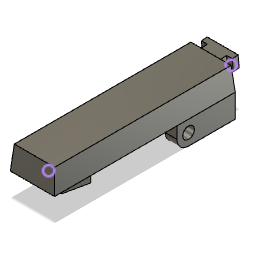
BlackKey (Autodesk Fusion 360 design; units mm, degrees)
Autodesk Fusion 360 part; units mm, degrees
note: some values were not read from the file. Set by a fixed rule: which sketch regions a step uses.
sketch "Sketch1" plane through (0, 0, 0) normal (0, 1, 0) x (1, 0, 0)
  line L0 (-2.54, 0) -> (7.112, 0)
  line L1 (7.112, 0) -> (7.112, -40.64)
  line L2 (7.112, -40.64) -> (-2.54, -40.64)
  line L3 (-2.54, -40.64) -> (-2.54, 0)
  dimension "d1" = 9.652
  dimension "d2" = 40.64
  constraint horizontal L0
  constraint vertical L1
  constraint horizontal L2
  constraint vertical L3
  measures "d1" distance of L0.start L0.end
  measures "d2" distance of L0.end L1.end
extrude "Extrude1" add sketch "Sketch1" along normal blind 5.08 draft -5
sketch "Sketch8" plane through (0, 0, 0) normal (0, -1, 0) x (1, 0, 0)
  line L0 (7.112, 40.64) -> (-2.54, 40.64)
  line L1 (-2.54, 40.64) -> (-2.54, 0)
  line L2 (-2.54, 0) -> (7.112, 0)
  line L3 (7.112, 0) -> (7.112, 40.64)
  line L4 (4.572, 2.54) -> (0, 2.54)
  line L5 (0, 2.54) -> (0, 38.1)
  line L6 (0, 38.1) -> (4.572, 38.1)
  line L7 (4.572, 38.1) -> (4.572, 2.54)
  line L8 (7.112, 0) -> (4.572, 0)
  line L9 (4.572, 0) -> (4.572, 12.7)
  line L10 (4.572, 12.7) -> (7.112, 12.7)
  line L11 (7.112, 12.7) -> (7.112, 0)
  line L12 (0, 0) -> (-2.54, 0)
  line L13 (-2.54, 0) -> (-2.54, 12.7)
  line L14 (-2.54, 12.7) -> (0, 12.7)
  line L15 (0, 12.7) -> (0, 0)
  line L16 (4.572, 0) -> (0, 0)
  line L17 (0, 0) -> (0, 2.54)
  line L18 (0, 2.54) -> (4.572, 2.54)
  line L19 (4.572, 2.54) -> (4.572, 0)
  dimension "d48" = 2.54
  dimension "d49" = 2.54
  dimension "d50" = 2.54
  dimension "d51" = 2.54
  dimension "d52" = 12.7
  dimension "d53" = 12.7
  constraint horizontal L4
  constraint vertical L5
  constraint horizontal L6
  constraint vertical L7
  constraint horizontal L8
  constraint vertical L9
  constraint horizontal L10
  constraint vertical L11
  constraint coincident L7 L9.end
  constraint coincident L2.end L3.start
  constraint horizontal L12
  constraint vertical L13
  constraint horizontal L14
  constraint vertical L15
  constraint coincident L1 L13.end
  constraint coincident L12.start L15.end
  constraint horizontal L16
  constraint vertical L17
  constraint horizontal L18
  constraint vertical L19
  measures "d48" distance of L0 L6
  measures "d49" distance of L2 L4
  measures "d50" distance of L1 L5
  measures "d51" distance of L3 L7
  measures "d52" distance of L2.end L10.end
  measures "d53" distance of L1.end L13.end
extrude "Extrude8" add sketch "Sketch8" along normal blind 5.08 contours L2 L3 L7 L8 L9 L10 L11 L19 | L1 L2 L5 L12 L13 L14 L15 L17
sketch "Sketch9" plane through (0, 0, 0) normal (0, 0.087156, -0.996195) x (-1, 0, 0)
  line L0 (2.0956, 5.0994) -> (-6.6676, 5.0994)
  line L1 (-6.6676, 5.0994) -> (-7.112, 0)
  line L2 (-7.112, 0) -> (-4.572, 0)
  line L3 (2.54, 0) -> (2.0956, 5.0994)
  line L4 (-6.8898, 2.5497) -> (-6.6676, 5.0994)
  line L5 (-6.6676, 5.0994) -> (2.0956, 5.0994)
  line L6 (2.0956, 5.0994) -> (2.3178, 2.5497)
  line L7 (-6.8898, 2.5497) -> (2.3178, 2.5497)
  line L8 (-4.572, 0) -> (0, 0)
  line L9 (0, 0) -> (2.54, 0)
  constraint midpoint L1 L4.start
  constraint coincident L0.end L1.start
  constraint coincident L0.start L3.end
  constraint midpoint L3 L6.end
extrude "Extrude9" add sketch "Sketch9" along normal blind 2.54 contours L0 L1 L3 L4 L5 L6 L7
sketch "Sketch13" plane through (7.112, 0, 0) normal (1, 0, 0) x (0, 0, -1)
  line L0 (-12.7, -5.08) -> (0, -5.08)
  line L1 (0, -5.08) -> (0, 0)
  line L2 (0, 0) -> (-12.7, 0)
  line L3 (-12.7, 0) -> (-12.7, -5.08)
  circle A0 centre (-10.16, -2.54) radius 1.27
  line L4 (0, -2.54) -> (-8.89, -2.54)
  line L5 (-11.43, -2.54) -> (-12.7, -2.54)
  line L6 (-10.16, -3.81) -> (-10.16, -5.08)
  constraint coincident L0 L6.end
  constraint midpoint L1 L4.start
  constraint coincident L3 L5.end
  constraint perpendicular L3 L4
  constraint coincident A0 L5.start
  constraint collinear L4 L5
  constraint coincident A0 L6.start
  constraint coincident A0 L4.end
extrude "Extrude12" cut sketch "Sketch13" against normal blind 20.32 contours A0
sketch "Sketch14" plane through (0, 0, 0) normal (0, -1, 0) x (1, 0, 0)
  line L0 (0, 12.7) -> (0, 0)
  line L1 (0, 0) -> (4.572, 0)
  line L2 (4.572, 0) -> (4.572, 12.7)
  line L3 (4.572, 12.7) -> (7.112, 12.7)
  line L4 (7.112, 12.7) -> (7.112, 40.64)
  line L5 (7.112, 40.64) -> (-2.54, 40.64)
  line L6 (-2.54, 40.64) -> (-2.54, 12.7)
  line L7 (-2.54, 12.7) -> (0, 12.7)
  line L8 (-2.54, 12.7) -> (0, 12.7)
  line L9 (-2.54, 40.64) -> (-2.54, 38.1)
  line L10 (0, 12.7) -> (0, 39.37)
  line L11 (0, 39.37) -> (4.9434, 39.37)
  line L12 (4.9434, 39.37) -> (4.572, 12.7)
  line L13 (0, 12.7) -> (4.572, 12.7)
  dimension "d72" = 2.54
  dimension "d73" = 2.54
  dimension "d74" = 26.67
  constraint coincident L6.end L7.start
  constraint perpendicular L6 L8
  constraint coincident L5.end L6.start
  constraint perpendicular L5 L9
  constraint coincident L0.start L7.end
  constraint perpendicular L8 L10
  constraint perpendicular L10 L11
  constraint coincident L2.end L3.start
  measures "d72" distance of L6.end L0.start
  measures "d73" distance of L5.end L9.end
  measures "d74" distance of L0.start L10.end
extrude "Extrude13" cut sketch "Sketch14" against normal blind 3.81 contours L10 L11 L12 L13
sketch "Sketch15" plane through (0, 0, 0) normal (0, -1, 0) x (1, 0, 0)
  line L0 (4.572, 12.7) -> (0, 12.7)
  line L1 (0, 12.7) -> (0, 0)
  line L2 (0, 0) -> (4.572, 0)
  line L3 (4.572, 0) -> (4.572, 12.7)
  line L4 (0, 0) -> (0, 2.54)
  line L5 (0, 2.54) -> (4.572, 2.54)
  line L6 (4.572, 2.54) -> (4.572, 12.7)
  line L7 (4.572, 12.7) -> (0, 12.7)
  line L8 (0, 12.7) -> (0, 2.54)
  dimension "d77" = 2.54
  constraint coincident L1.end L2.start
  constraint perpendicular L2 L4
  constraint horizontal L5
  constraint vertical L6
  constraint horizontal L7
  constraint vertical L8
  constraint coincident L0.start L3.end
  measures "d77" distance of L1.end L4.end
extrude "Extrude14" cut sketch "Sketch15" against normal blind 2.54 contours L0 L1 L3 L5 L6 L7 L8
extrude "Extrude15" cut 1 faces at (1.524, 2.54, 5.9267) along direction (0, 1, 0) blind 1.27
sketch "Sketch16" plane through (7.112, 0, 0) normal (1, 0, 0) x (0, 0, -1)
  circle A0 centre (-10.16, -2.54) radius 1.27
  line L0 (0, 0) -> (-12.7, 0)
  line L1 (-12.7, 0) -> (-12.7, -5.08)
  line L2 (-12.7, -5.08) -> (0, -5.08)
  line L3 (0, -5.08) -> (0, 0)
  line L4 (-12.7, -2.54) -> (-12.7, -5.08)
  line L5 (-10.16, -5.08) -> (-12.7, -5.08)
  arc A1 (-12.7, -2.54) -> (-10.16, -5.08) centre (-10.16, -2.54) ccw
  constraint concentric A0 A1
  constraint tangent L2 A1
  constraint midpoint L1 L4.start
  constraint coincident L1.end L2.start
  constraint tangent L5 A1
extrude "Extrude16" cut sketch "Sketch16" against normal blind 10.414 contours L1 L2 L4 L5 A1
sketch "Sketch17" plane through (0, 0, 0) normal (0, -1, 0) x (1, 0, 0)
  line L0 (0, 12.7) -> (0, 39.37)
  line L1 (0, 39.37) -> (4.9434, 39.37)
  line L2 (4.9434, 39.37) -> (4.572, 12.7)
  line L3 (4.572, 12.7) -> (7.112, 12.7)
  line L4 (7.112, 12.7) -> (7.112, 40.64)
  line L5 (7.112, 40.64) -> (-2.54, 40.64)
  line L6 (-2.54, 40.64) -> (-2.54, 12.7)
  line L7 (-2.54, 12.7) -> (0, 12.7)
  line L8 (0, 39.37) -> (-1.27, 39.37)
  line L9 (-1.27, 39.37) -> (-1.27, 12.7)
  line L10 (-1.27, 12.7) -> (0, 12.7)
  line L11 (0, 12.7) -> (0, 39.37)
  constraint horizontal L8
  constraint vertical L9
  constraint horizontal L10
  constraint vertical L11
  constraint midpoint L7 L9.end
  constraint coincident L0.end L1.start
extrude "Extrude17" cut sketch "Sketch17" against normal blind 3.81 contours L0 L7 L8 L9 L10 L11
extrude "Extrude18" cut 1 faces at (4.8196, 1.27, 30.48) along direction (0.999903, 0, -0.013923) blind 1.27
sketch "Sketch18" plane through (0, 0, 0) normal (0, 1, 0) x (1, 0, 0)
extrude "Extrude19" add 1 faces at (1.2245, 3.81, 30.48) along direction (0, -1, 0) blind 3.81
sketch "Sketch19" plane through (0, 5.08, 0.4444) normal (0, 0.996195, 0.087156) x (1, 0, 0)
  line L0 (-2.0956, 0) -> (6.6676, 0)
  line L1 (6.6676, 0) -> (6.6676, 2.54)
  line L2 (6.6676, 2.54) -> (-2.0956, 2.54)
  line L3 (-2.0956, 2.54) -> (-2.0956, 0)
  line L4 (2.286, 2.54) -> (-1.0795, 2.54)
  line L5 (2.286, 2.54) -> (5.6642, 2.54)
  line L6 (-1.0795, 2.54) -> (-1.0795, 1.27)
  line L7 (-1.0795, 1.27) -> (0.1905, 1.27)
  line L8 (0.1905, 1.27) -> (0.1905, 0)
  line L9 (5.6642, 2.54) -> (5.6642, 1.27)
  line L10 (5.6642, 1.27) -> (4.3942, 1.27)
  line L11 (4.3942, 1.27) -> (4.3942, 0)
  line L12 (0.1905, 0) -> (4.3942, 0)
  line L13 (4.3942, 0) -> (7.366, 0)
  line L14 (7.366, 0) -> (7.366, 2.54)
  line L15 (7.366, 2.54) -> (5.6642, 2.54)
  line L16 (-1.0795, 2.54) -> (-2.794, 2.54)
  line L17 (-2.794, 2.54) -> (-2.794, 0)
  line L18 (-2.794, 0) -> (0.1905, 0)
  dimension "d91" = 3.3655
  dimension "d92" = 3.3782
  dimension "d93" = 1.27
  dimension "d94" = 1.27
  dimension "d95" = 1.27
  dimension "d96" = 1.27
  constraint midpoint L2 L4.start
  constraint parallel L2 L4
  constraint parallel L2 L5
  constraint perpendicular L2 L6
  constraint perpendicular L6 L7
  constraint coincident L0 L8.end
  constraint perpendicular L0 L8
  constraint perpendicular L5 L9
  constraint perpendicular L9 L10
  constraint coincident L0 L11.end
  constraint perpendicular L0 L11
  constraint perpendicular L1 L13
  constraint perpendicular L0 L14
  constraint perpendicular L6 L16
  constraint perpendicular L16 L17
  constraint perpendicular L8 L18
  measures "d91" distance of L4.start L4.end
  measures "d92" distance of L4.start L5.end
  measures "d93" distance of L4.end L6.end
  measures "d94" distance of L6.end L7.end
  measures "d95" distance of L5.end L9.end
  measures "d96" distance of L9.end L10.end
extrude "Extrude20" cut sketch "Sketch19" against normal blind 5.08 contours L0 L2 L3 L6 L7 L8 L16 L18 | L3 L16 L17 L18 | L0 L1 L2 L9 L10 L11 L13 L15 | L1 L13 L14 L15
sketch "Sketch21" plane through (7.058, 0.6175, 0) normal (0.996195, 0.087156, 0) x (0, 0, -1)
  line L0 (-40.1956, 4.4796) -> (-40.64, -0.6199)
  line L1 (-40.64, -0.6199) -> (-12.7, -0.6199)
  line L2 (-12.7, -0.6199) -> (0, -0.6199)
  line L3 (0, -0.6199) -> (-0.4444, 4.4796)
sketch "Sketch22" plane through (0, 0, 0) normal (0, -1, 0) x (1, 0, 0)
  line L0 (4.572, 12.7) -> (7.112, 12.7)
  line L1 (7.112, 12.7) -> (7.112, 40.64)
  line L2 (7.112, 40.64) -> (-2.54, 40.64)
  line L3 (-2.54, 40.64) -> (-2.54, 12.7)
  line L4 (-2.54, 12.7) -> (0, 12.7)
  line L5 (0, 12.7) -> (0, 0)
  line L6 (0, 0) -> (4.572, 0)
  line L7 (4.572, 0) -> (4.572, 12.7)
  line L8 (-2.54, 40.64) -> (-2.54, 33.02)
  line L9 (7.112, 33.02) -> (5.461, 33.02)
  line L10 (2.286, 36.195) -> (5.461, 36.195)
  line L11 (5.461, 36.195) -> (-0.889, 36.195)
  line L12 (-0.889, 36.195) -> (-0.889, 29.845)
  line L13 (-0.889, 29.845) -> (5.461, 29.845)
  line L14 (5.461, 29.845) -> (5.461, 36.195)
  line L15 (2.286, 40.64) -> (2.286, 36.195)
  line L16 (2.286, 29.845) -> (2.286, 0)
  dimension "d100" = 3.175
  dimension "d101" = 6.35
  dimension "d102" = 6.35
  constraint midpoint L2 L15.start
  constraint midpoint L6 L16.end
  constraint coincident L2.end L3.start
  constraint coincident L3 L8.end
  constraint perpendicular L2 L8
  constraint coincident L1 L9.start
  constraint perpendicular L9 L15
  constraint perpendicular L10 L15
  constraint horizontal L11
  constraint vertical L12
  constraint horizontal L13
  constraint vertical L14
  constraint collinear L15 L16
  constraint coincident L13 L16.start
  constraint coincident L14 L9.end
  measures "d100" distance of L10.start L10.end
  measures "d101" distance of L10.end L11.end
  measures "d102" distance of L10.end L13.end
extrude "Extrude21" add sketch "Sketch22" along normal blind 5.08 contours L10 L11 L12 L13 L14
sketch "Sketch23" plane through (7.058, 0.6175, 0) normal (0.996195, 0.087156, 0) x (0, 0, -1)
sketch "Sketch24" plane through (5.461, 0, 0) normal (1, 0, 0) x (0, 0, -1)
  line L0 (-29.845, 0) -> (-36.195, 0)
  line L1 (-36.195, 0) -> (-36.195, -5.08)
  line L2 (-36.195, -5.08) -> (-29.845, -5.08)
  line L3 (-29.845, -5.08) -> (-29.845, 0)
  line L4 (-29.845, 0) -> (-29.845, -3.024)
  line L5 (-36.195, 0) -> (-36.195, -1.9064)
  line L6 (-36.195, -1.9064) -> (-29.845, -3.024)
  dimension "d105" = 3.024
  dimension "d106" = 1.9064
  constraint coincident L0.start L3.end
  constraint perpendicular L2 L4
  constraint coincident L0.end L1.start
  constraint perpendicular L0 L5
  measures "d105" distance of L0.start L4.end
  measures "d106" distance of L0.end L5.end
extrude "Extrude22" cut sketch "Sketch24" against normal blind 6.35 contours L1 L2 L3 L6
extrude "Extrude23" cut 1 faces at (3.7465, 1.6933, 40.4919) along direction (0, -0.087156, -0.996195) blind 1.27
sketch "Sketch26" plane through (0, 1.5515, -0.1357) normal (0, -0.996195, 0.087156) x (1, 0, 0)
  line L0 (6.6676, 40.4854) -> (-2.0956, 40.4854)
  line L1 (-2.0956, 40.4854) -> (-2.0956, 39.2154)
  line L2 (-2.0956, 39.2154) -> (6.6676, 39.2154)
  line L3 (6.6676, 39.2154) -> (6.6676, 40.4854)
extrude "Extrude24" cut sketch "Sketch26" against normal blind 1.27
sketch "Sketch27" plane through (-2.2145, 0.1923, -0.0168) normal (0.996223, -0.086496, 0.007567) x (0.007596, 0, -0.999971)
  line L0 (-40.6581, -0.193) -> (-39.3832, -0.193)
  line L1 (-39.3832, -0.193) -> (-38.9452, 4.795)
  line L2 (-38.9452, 4.795) -> (-40.2103, 4.9061)
  line L3 (-40.2103, 4.9061) -> (-40.6581, -0.193)
  line L4 (-38.9348, 4.9137) -> (-40.2103, 4.9061)
  line L5 (-40.2103, 4.9061) -> (-40.6581, -0.193)
  line L6 (-40.6581, -0.193) -> (-39.37, -0.193)
  line L7 (-39.37, -0.193) -> (-38.9348, 4.9137)
  constraint coincident L2.end L3.start
  constraint perpendicular L2 L5
  constraint parallel L0 L6
extrude "Extrude25" cut sketch "Sketch27" against normal blind 2.794 contours L0 L1 L2 L3 L5 L6 | L2 L4 L7
extrude "Extrude26" cut 1 faces at (-2.5367, 0.0003, 39.7901) along direction (-0.086494, -0.996252, -0.000657) blind 0.2286
sketch "Sketch30" plane through (7.058, 0.6175, 0) normal (0.996195, 0.087156, 0) x (0, 0, -1)
  line L0 (-38.9382, 4.4704) -> (-39.37, -0.635)
  line L1 (-39.37, -0.635) -> (-40.64, -0.635)
  line L2 (-40.64, -0.635) -> (-40.6939, 4.507)
  line L3 (-40.6939, 4.507) -> (-38.9382, 4.4704)
  constraint horizontal L1
extrude "Extrude27" cut sketch "Sketch30" against normal blind 0.254
equation "d91 = ( 0.265 / 2 ) * 1 in"
equation "d105 = 0.06 in + 1.5 mm"
equation "d106 = 0.016 in + 1.5 mm"
